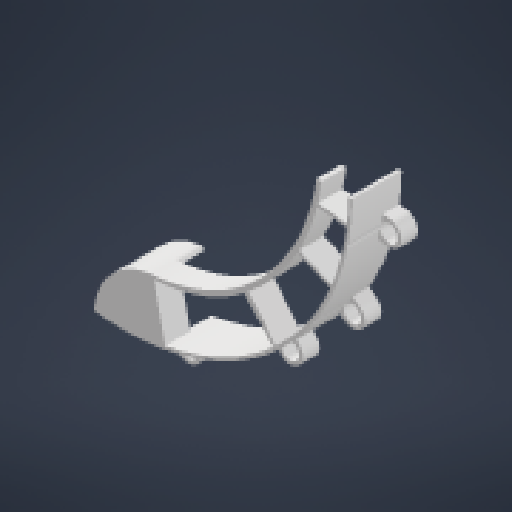
# Autodesk Inventor part: HalfFilterWall2
Saved by Autodesk Inventor 2026 (Build 300175050, 175E)
## iProperties
Created: 2026-05-05
Part Number: HalfFilterWall2
Material: Generic
Document SubType Name: Modeling
Designer: sniel
Density: 1 g/cm^3
Appearance: Default
Author: sniel
Autodesk Inventor part; units mm, degrees
ref_plane "YZ Plane" through (0, 0, 0) normal (1, 0, 0) x (0, 1, 0)
ref_plane "XZ Plane" through (0, 0, 0) normal (0, 1, 0) x (-1, 0, 0)
ref_plane "XY Plane" through (0, 0, 0) normal (0, 0, 1) x (1, 0, 0)
sketch "Sketch1" plane through (0, 0, 0) normal (0, 0, 1) x (1, 0, 0)
  arc A0 (23.689125, 20.041184) -> (18.254395, 20.887332) centre (0, -114.235526) ccw
  arc A1 (18.254395, 20.887332) -> (1.007395, 22.112112) centre (0, -114.119689) ccw
  arc A2 (1.007395, 22.112112) -> (0, 21.11214) centre (1, 21.11214) ccw
  line L0 (0, 21.11214) -> (0, 20.996303)
  arc A3 (0, 20.996303) -> (0.992605, 19.99633) centre (1, 20.996303) ccw
  arc A4 (16.894539, 18.932605) -> (0.992605, 19.99633) centre (0, -114.235526) ccw
  arc A5 (17.756944, 17.787789) -> (16.894539, 18.932605) centre (16.768682, 17.940556) ccw
  line L1 (17.756944, 17.787789) -> (16.790242, 11.534134)
  arc A6 (15.60857, 10.705783) -> (16.790242, 11.534134) centre (15.80198, 11.686902) ccw
  arc A7 (15.60857, 10.705783) -> (1.079217, 12.70838) centre (-9, -114.127341) ccw
  arc A8 (1.079217, 12.70838) -> (0, 11.711522) centre (1, 11.711522) ccw
  line L2 (0, 11.711522) -> (0, 11.060813)
  arc A9 (0, 11.060813) -> (0.916491, 10.064306) centre (1, 11.060813) ccw
  arc A10 (115.231581, -113.243479) -> (0.916491, 10.064306) centre (-9.5, -114.235526) ccw
  arc A11 (118.232397, -113.228461) -> (114.566766, -83.793446) centre (-9, -114.127341) ccw
  arc A12 (115.32455, -82.578069) -> (114.566766, -83.793446) centre (115.537931, -83.555038) ccw
  line L3 (115.32455, -82.578069) -> (128.714541, -79.65355)
  arc A13 (129.895591, -80.378296) -> (128.714541, -79.65355) centre (128.927921, -80.630519) ccw
  arc A14 (134.231856, -113.242921) -> (129.895591, -80.378296) centre (0, -114.235526) ccw
  arc A15 (134.231856, -113.242921) -> (135.231829, -114.235526) centre (135.231829, -113.235526) ccw
  line L4 (135.231829, -114.235526) -> (135.232636, -114.235526)
  arc A16 (135.232636, -114.235526) -> (136.232614, -113.228988) centre (135.232636, -113.235526) ccw
  arc A17 (136.232614, -113.228988) -> (135.007021, -95.865294) centre (0, -114.119689) ccw
  line L5 (135.007021, -95.865294) -> (135.104981, -95.849292)
  arc A18 (135.104981, -95.849292) -> (134.27671, -90.546401) centre (0, -114.235526) ccw
  arc A19 (133.568756, -86.834851) -> (134.27671, -90.546401) centre (138.734281, -87.772854) ccw
  arc A20 (133.568756, -86.834851) -> (132.332251, -81.378487) centre (0, -114.235526) ccw
  line L6 (132.332251, -81.378487) -> (132.247295, -81.397042)
  arc A21 (132.247295, -81.397042) -> (116.651364, -43.745136) centre (0, -114.119689) ccw
  line L7 (116.651364, -43.745136) -> (116.697607, -43.715472)
  arc A22 (116.697607, -43.715472) -> (113.822576, -39.163356) centre (0, -114.235526) ccw
  arc A23 (111.698714, -36.038295) -> (113.822576, -39.163356) centre (116.811886, -34.84751) ccw
  arc A24 (111.698714, -36.038295) -> (108.408382, -31.537085) centre (0, -114.235526) ccw
  line L8 (108.408382, -31.537085) -> (108.372186, -31.563116)
  arc A25 (108.372186, -31.563116) -> (82.556573, -5.747503) centre (0, -114.119689) ccw
  line L9 (82.556573, -5.747503) -> (82.569791, -5.729124)
  arc A26 (82.569791, -5.729124) -> (78.197231, -2.536812) centre (0, -114.235526) ccw
  arc A27 (75.07217, -0.41295) -> (78.197231, -2.536812) centre (79.388016, 2.57636) ccw
  arc A28 (75.07217, -0.41295) -> (70.382977, 2.544807) centre (0, -114.235526) ccw
  line L10 (70.382977, 2.544807) -> (70.374553, 2.531675)
  arc A29 (70.374553, 2.531675) -> (32.722647, 18.127606) centre (0, -114.119689) ccw
  line L11 (32.722647, 18.127606) -> (32.723148, 18.129897)
  arc A30 (32.723148, 18.129897) -> (27.400675, 19.33323) centre (0, -114.235526) ccw
  arc A31 (23.689125, 20.041184) -> (27.400675, 19.33323) centre (26.462672, 24.498755) ccw
  arc A32 (113.560126, -79.952698) -> (76.239267, -19.664872) centre (-9, -114.127341) ccw
  arc A33 (76.174631, -18.243916) -> (76.239267, -19.664872) centre (76.9092, -18.92245) ccw
  line L12 (76.174631, -18.243916) -> (83.492463, -10.321763)
  arc A34 (84.859198, -10.225464) -> (83.492463, -10.321763) centre (84.227031, -11.000297) ccw
  arc A35 (128.819481, -76.490091) -> (84.859198, -10.225464) centre (0, -114.235526) ccw
  arc A36 (128.073209, -77.748248) -> (128.819481, -76.490091) centre (127.859828, -76.771279) ccw
  line L13 (128.073209, -77.748248) -> (114.73676, -80.661074)
  arc A37 (113.560126, -79.952698) -> (114.73676, -80.661074) centre (114.52338, -79.684104) ccw
  line L14 (18.728755, 11.004204) -> (19.737656, 17.530849)
  arc A38 (20.881477, 18.365908) -> (19.737656, 17.530849) centre (20.725918, 17.378082) ccw
  arc A39 (81.689945, -7.718254) -> (20.881477, 18.365908) centre (0, -114.235526) ccw
  arc A40 (81.815957, -9.190298) -> (81.689945, -7.718254) centre (81.081388, -8.511764) ccw
  line L15 (81.815957, -9.190298) -> (74.632091, -16.967423)
  arc A41 (73.251075, -17.051848) -> (74.632091, -16.967423) centre (73.897522, -16.288889) ccw
  arc A42 (73.251075, -17.051848) -> (19.493078, 9.876833) centre (-9, -114.127341) ccw
  arc A43 (18.728755, 11.004204) -> (19.493078, 9.876833) centre (19.717017, 10.851436) ccw
  circle A44 centre (26.462672, -252.969807) radius 5.25
  circle A45 centre (79.388016, -231.047412) radius 5.25
  circle A46 centre (138.734281, -140.698198) radius 5.25
  circle A47 centre (116.811886, -193.623542) radius 5.25
  line L16 (70.374553, -230.886891) -> (73.075233, -235.096951)
  arc A48 (73.075233, -235.096951) -> (85.476933, -226.668474) centre (79.388016, -231.047412) ccw
  line L17 (85.476933, -226.668474) -> (82.556573, -222.607712)
  arc A49 (82.556573, -222.607712) -> (108.372186, -196.792099) centre (0, -114.235526) ccw
  line L18 (108.372186, -196.792099) -> (112.432948, -199.712459)
  arc A50 (112.432948, -199.712459) -> (120.861425, -187.310759) centre (116.811886, -193.623542) ccw
  line L19 (120.861425, -187.310759) -> (116.651364, -184.610079)
  arc A51 (116.651364, -184.610079) -> (132.247295, -146.958173) centre (0, -114.235526) ccw
  line L20 (132.247295, -146.958173) -> (137.133926, -148.025467)
  arc A52 (137.133926, -148.025467) -> (139.943419, -133.296307) centre (138.734281, -140.698198) ccw
  line L21 (139.943419, -133.296307) -> (135.007021, -132.489921)
  arc A53 (135.007021, -132.489921) -> (136.235526, -114.235526) centre (0, -114.235526) ccw
  line L22 (136.235526, -114.235526) -> (134.235526, -114.235526)
  line L23 (0, -248.471052) -> (0, -250.471052)
  arc A54 (19.060781, -254.178945) -> (33.789941, -251.369452) centre (26.462672, -252.969807) ccw
  line L24 (33.789941, -251.369452) -> (32.722647, -246.482821)
  arc A55 (32.722647, -246.482821) -> (70.374553, -230.886891) centre (0, -114.235526) ccw
  arc A56 (69.722359, -193.081889) -> (115.100471, -114.235526) centre (-4.40842, -97.9364) ccw
  line L25 (118.110658, -114.235526) -> (115.100471, -114.235526)
  line L26 (133.484281, -128.417314) -> (112.842728, -126.224291)
  line L27 (133.484281, -128.417314) -> (133.258174, -130.404492)
  line L28 (115.9197, -126.551198) -> (115.452307, -128.495817)
  line L29 (115.452307, -128.495817) -> (133.258174, -130.404492)
  line L30 (124.355241, -164.782045) -> (123.588357, -166.629175)
  line L31 (123.588357, -166.629175) -> (103.639403, -158.346853)
  line L32 (124.355241, -164.782045) -> (104.606006, -156.582642)
  line L33 (89.213784, -214.535462) -> (90.698228, -213.195154)
  line L34 (90.698228, -213.195154) -> (72.751914, -190.641952)
  line L35 (89.213784, -214.535462) -> (69.722359, -193.081889)
  circle A57 centre (-138.734281, -140.698198) radius 5.25
  circle A58 centre (-116.811886, -193.623542) radius 5.25
  circle A59 centre (-26.462672, -252.969807) radius 5.25
  circle A60 centre (-79.388016, -231.047412) radius 5.25
  line L36 (-116.651364, -184.610079) -> (-120.861425, -187.310759)
  arc A61 (-120.861425, -187.310759) -> (-112.432948, -199.712459) centre (-116.811886, -193.623542) ccw
  line L37 (-112.432948, -199.712459) -> (-108.372186, -196.792099)
  arc A62 (-108.372186, -196.792099) -> (-82.556573, -222.607712) centre (0, -114.235526) ccw
  line L38 (-82.556573, -222.607712) -> (-85.476933, -226.668474)
  arc A63 (-85.476933, -226.668474) -> (-73.075233, -235.096951) centre (-79.388016, -231.047412) ccw
  line L39 (-73.075233, -235.096951) -> (-70.374553, -230.886891)
  arc A64 (-70.374553, -230.886891) -> (-32.722647, -246.482821) centre (0, -114.235526) ccw
  line L40 (-32.722647, -246.482821) -> (-33.789941, -251.369452)
  arc A65 (-33.789941, -251.369452) -> (-19.060781, -254.178945) centre (-26.462672, -252.969807) ccw
  line L41 (-19.060781, -254.178945) -> (-18.254395, -249.242547)
  arc A66 (-18.254395, -249.242547) -> (0, -250.471052) centre (0, -114.235526) ccw
  line L42 (0, -250.471052) -> (0, -248.471052)
  arc A67 (-134.235526, -114.235526) -> (0, -248.471052) centre (0, -114.235526) ccw
  line L43 (-134.235526, -114.235526) -> (-136.235526, -114.235526)
  arc A68 (-136.235526, -114.235526) -> (-135.007021, -132.489921) centre (0, -114.235526) ccw
  line L44 (-135.007021, -132.489921) -> (-139.943419, -133.296307)
  arc A69 (-139.943419, -133.296307) -> (-137.133926, -148.025467) centre (-138.734281, -140.698198) ccw
  line L45 (-137.133926, -148.025467) -> (-132.247295, -146.958173)
  arc A70 (-132.247295, -146.958173) -> (-116.651364, -184.610079) centre (0, -114.235526) ccw
  arc A71 (22.567907, -246.560376) -> (27.724702, -245.576751) centre (26.462672, -252.969807) ccw
  arc A72 (22.567907, -246.560376) -> (134.235526, -114.235526) centre (0, -114.235526) ccw
  line L46 (0, -248.471052) -> (0, -216.471052)
  line L47 (0, -216.471052) -> (0, -214.471052)
  circle A73 centre (0, -250.471052) radius 16
  line L48 (26.462672, -252.969807) -> (22.567907, -246.560376)
  circle A74 centre (22.567907, -246.560376) radius 32
  arc A75 (16.034625, -215.234409) -> (-15.97239, -249.531503) centre (24.34296, -255.071453) ccw
  line L49 (22.567907, -246.560376) -> (16.034625, -215.234409)
  line L50 (16.034625, -215.234409) -> (15.626295, -213.276536)
  arc A76 (15.626295, -213.276536) -> (-18.254395, -249.242547) centre (20.539292, -251.84582) ccw
  arc A77 (71.73985, -195.302476) -> (118.110658, -114.235526) centre (-2.270449, -99.172443) ccw
  arc A78 (15.626295, -213.276536) -> (69.722359, -193.081889) centre (7.954113, -110.173035) ccw
  arc A79 (16.034625, -215.234409) -> (71.73985, -195.302476) centre (13.040909, -119.059964) ccw
  line L51 (15.626295, -213.276536) -> (17.619252, -213.108837)
  line L52 (22.567907, -246.560376) -> (24.53688, -246.209455)
  line L53 (24.53688, -246.209455) -> (17.619252, -213.108837)
  point P0 (74.632091, -193.004777)
  point P1 (33.789941, -244.148637)
  point P2 (36.843345, -243.315905)
  point P3 (33.789941, -251.369452)
  point P4 (-15.213711, -245.516964)
  point P5 (24.373197, -214.61134)
  point P6 (19.060781, -254.178945)
  point P7 (33.789941, -251.369452)
  point P8 (18.045983, -215.150731)
  point P9 (17.991354, -214.88933)
  point P10 (22.567907, -246.560376)
  dimension "d68" = 32
  dimension "d69" = 64
  dimension "d54" = 2
  dimension "d55" = 2
  dimension "d56" = 2
  dimension "d57" = 2
  dimension "d66" = 32
  dimension "d67" = 2
  dimension "d70" = 2
  dimension "d71" = 2
  dimension "d72" = 2
  constraints: 148 point on circle, 108 end point, 77 centre point, 4 point on line, 3 coincident, 1 concentric, 1 horizontal, 1 perpendicular, 1 tangent, 21 other
  measures "d54" distance of L26.start L27.end
  measures "d55" distance of L28.start L28.end
  measures "d56" distance of L30.start L30.end
  measures "d57" distance of L33.start L33.end
  measures "d66" distance of L23.start L46.end
  measures "d67" distance of L46.end L47.end
  measures "d70" distance of L49.end L50.end
  measures "d71" distance of L50.end L51.end
  measures "d72" distance of L49.start L52.end
extrude "Extrusion1" add sketch "Sketch1" along normal blind 30 contours A55 A74 A72 L22 A53 L21 A52 L20 A51 L19 A50 L18 A49 L17 A48 L16 | A55 L24 A71 A72 A74 | A54 A71 A72 | L35 A77 L34 L33 | A74 L53 A78 L35 A79 | A66 A76 A67 A73 | A72 L52 | L52 L49 A79 L53 | L35 A56 L34 A77 | L53 A79 A74 | A74 L50 A78 L53 | A67 A76 L46 A75 A73 | L34 A56 L26 L28 A77 | L31 A77 L32 L30 | A75 L46 A76 L50 | A56 L25 A77 L26 | L29 A77 L26 L27 | A77 L28 picked at (17.804356, -215.074453)
sketch "Sketch9" plane through (0, 0, 0) normal (0, 0, -1) x (-1, 0, 0)
  line L0 (-136.235526, -114.235526) -> (-134.235526, -114.235526)
  arc A0 (-134.235526, -114.235526) -> (-133.484281, -128.417314) centre (0, -114.235526) ccw
  arc A1 (-90.698228, -213.195154) -> (-89.213784, -214.535462) centre (0, -114.235526) ccw
  line L1 (-71.73985, -195.302476) -> (-89.213784, -214.535462)
  line L2 (-89.213784, -214.535462) -> (-90.698228, -213.195154)
  line L3 (-90.698228, -213.195154) -> (-74.632091, -193.004777)
  line L4 (-115.452307, -128.495817) -> (-133.258174, -130.404492)
  line L5 (-133.258174, -130.404492) -> (-133.484281, -128.417314)
  line L6 (-133.484281, -128.417314) -> (-115.9197, -126.551198)
  line L7 (-118.110658, -114.235526) -> (-115.100471, -114.235526)
  arc A2 (-115.100471, -114.235526) -> (-69.722359, -193.081889) centre (4.40842, -97.9364) ccw
  line L8 (-33.789941, -251.369452) -> (-32.722647, -246.482821)
  arc A3 (-70.374553, -230.886891) -> (-32.722647, -246.482821) centre (0, -114.235526) ccw
  line L9 (-70.374553, -230.886891) -> (-73.075233, -235.096951)
  arc A4 (-85.476933, -226.668474) -> (-73.075233, -235.096951) centre (-79.388016, -231.047412) ccw
  line L10 (-85.476933, -226.668474) -> (-82.556573, -222.607712)
  arc A5 (-108.372186, -196.792099) -> (-82.556573, -222.607712) centre (0, -114.235526) ccw
  line L11 (-108.372186, -196.792099) -> (-112.432948, -199.712459)
  arc A6 (-120.861425, -187.310759) -> (-112.432948, -199.712459) centre (-116.811886, -193.623542) ccw
  line L12 (-120.861425, -187.310759) -> (-116.651364, -184.610079)
  arc A7 (-132.247295, -146.958173) -> (-116.651364, -184.610079) centre (0, -114.235526) ccw
  line L13 (-132.247295, -146.958173) -> (-137.133926, -148.025467)
  arc A8 (-139.943419, -133.296307) -> (-137.133926, -148.025467) centre (-138.734281, -140.698198) ccw
  line L14 (-139.943419, -133.296307) -> (-135.007021, -132.489921)
  arc A9 (-136.235526, -114.235526) -> (-135.007021, -132.489921) centre (0, -114.235526) ccw
  circle A10 centre (-116.811886, -193.623542) radius 5.25
  circle A11 centre (-138.734281, -140.698198) radius 5.25
  circle A12 centre (-79.388016, -231.047412) radius 5.25
  circle A13 centre (0, -114.235526) radius 134.235526
  arc A14 (-118.110658, -114.235526) -> (-115.9197, -126.551198) centre (2.270449, -99.172443) ccw
  arc A15 (-103.639403, -158.346853) -> (-74.632091, -193.004777) centre (2.270449, -99.172443) ccw
  arc A16 (-133.258174, -130.404492) -> (-124.355241, -164.782045) centre (0, -114.235526) ccw
  arc A17 (-89.213784, -214.535462) -> (-24.53688, -246.209455) centre (0, -114.235526) ccw
  arc A18 (-133.484281, -128.417314) -> (-133.258174, -130.404492) centre (0, -114.235526) ccw
  arc A19 (-124.355241, -164.782045) -> (-123.588357, -166.629175) centre (0, -114.235526) ccw
  arc A20 (-33.789941, -251.369452) -> (-22.567907, -246.560376) centre (-26.462672, -252.969807) ccw
  arc A21 (-69.722359, -193.081889) -> (-15.626295, -213.276536) centre (-7.954113, -110.173035) ccw
  arc A22 (18.254395, -249.242547) -> (-15.626295, -213.276536) centre (-20.539292, -251.84582) ccw
  arc A23 (15.97239, -249.531503) -> (18.254395, -249.242547) centre (0, -114.235526) ccw
  arc A24 (15.97239, -249.531503) -> (15.213711, -245.516964) centre (0, -250.471052) ccw
  arc A25 (15.213711, -245.516964) -> (-16.034625, -215.234409) centre (-24.34296, -255.071453) ccw
  arc A26 (-17.991354, -214.88933) -> (-24.373197, -214.61134) centre (-22.567907, -246.560376) ccw
  arc A27 (-71.73985, -195.302476) -> (-24.373197, -214.61134) centre (-13.040909, -119.059964) ccw
  line L15 (-103.639403, -158.346853) -> (-123.588357, -166.629175)
  line L16 (-123.588357, -166.629175) -> (-124.355241, -164.782045)
  line L17 (-124.355241, -164.782045) -> (-104.606006, -156.582642)
  arc A28 (-115.452307, -128.495817) -> (-104.606006, -156.582642) centre (2.270449, -99.172443) ccw
  circle A29 centre (-24.34296, -255.071453) radius 40.460125
  arc A30 (-71.73985, -195.302476) -> (-24.373197, -214.61134) centre (-13.040909, -119.059964) ccw
  arc A31 (-69.722359, -193.081889) -> (-15.626295, -213.276536) centre (-7.954113, -110.173035) ccw
  line L18 (-24.373197, -214.61134) -> (-15.626295, -213.276536)
  line L19 (-16.034625, -215.234409) -> (-22.567907, -246.560376)
  arc A32 (-123.588357, -166.629175) -> (-90.698228, -213.195154) centre (0, -114.235526) ccw
  line L20 (-24.53688, -246.209455) -> (-17.991354, -214.88933)
  point P0 (0, 0)
  point P1 (-24.53688, -246.209455)
  point P2 (-133.484281, -128.417314)
  point P3 (-133.258174, -130.404492)
  point P4 (-124.355241, -164.782045)
  point P5 (-22.567907, -246.560376)
  point P6 (-89.213784, -214.535462)
  point P7 (-90.698228, -213.195154)
  point P8 (-133.484281, -128.417314)
  point P9 (-124.355241, -164.782045)
  point P10 (15.730389, -247.546183)
  point P11 (18.068997, -247.249389)
  point P12 (-22.567907, -246.560376)
  point P13 (-24.53688, -246.209455)
  point P14 (15.418073, -247.582665)
  point P15 (-18.036598, -215.105825)
  constraints: 2 coincident, 2 end point, 1 centre point, 3 other
extrude "Extrusion8" cut sketch "Sketch9" against normal blind 15 contours A13 A22 A21 A2 L7 A14 L6 A0 | L6 A14 L7 A2 A21 L18 A27 L1 L2 L3 A15 L15 L16 L17 A28 L4 L5 | L4 A28 L17 A13 | L16 A13 | A13 A29 L19 A25 A24 | L15 A15 L3 A13 | A13 L19 A29 | A29 A13 L1 A27 | A26 L20 A29 | A29 L20 A13 | A13 L20 A29 L19
sketch "Sketch10" plane through (0, 0, 30) normal (0, 0, 1) x (1, 0, 0)
  line L0 (136.235526, -114.235526) -> (134.235526, -114.235526)
  line L1 (71.73985, -195.302476) -> (89.213784, -214.535462)
  line L2 (89.213784, -214.535462) -> (90.698228, -213.195154)
  line L3 (90.698228, -213.195154) -> (74.632091, -193.004777)
  line L4 (115.452307, -128.495817) -> (133.258174, -130.404492)
  line L5 (133.258174, -130.404492) -> (133.484281, -128.417314)
  line L6 (133.484281, -128.417314) -> (115.9197, -126.551198)
  arc A0 (115.9197, -126.551198) -> (118.110658, -114.235526) centre (-2.270449, -99.172443) ccw
  line L7 (118.110658, -114.235526) -> (115.100471, -114.235526)
  arc A1 (69.722359, -193.081889) -> (115.100471, -114.235526) centre (-4.40842, -97.9364) ccw
  line L8 (33.789941, -251.369452) -> (32.722647, -246.482821)
  arc A2 (32.722647, -246.482821) -> (70.374553, -230.886891) centre (0, -114.235526) ccw
  line L9 (70.374553, -230.886891) -> (73.075233, -235.096951)
  arc A3 (73.075233, -235.096951) -> (85.476933, -226.668474) centre (79.388016, -231.047412) ccw
  line L10 (85.476933, -226.668474) -> (82.556573, -222.607712)
  arc A4 (82.556573, -222.607712) -> (108.372186, -196.792099) centre (0, -114.235526) ccw
  line L11 (108.372186, -196.792099) -> (112.432948, -199.712459)
  arc A5 (112.432948, -199.712459) -> (120.861425, -187.310759) centre (116.811886, -193.623542) ccw
  line L12 (120.861425, -187.310759) -> (116.651364, -184.610079)
  arc A6 (116.651364, -184.610079) -> (132.247295, -146.958173) centre (0, -114.235526) ccw
  line L13 (132.247295, -146.958173) -> (137.133926, -148.025467)
  arc A7 (137.133926, -148.025467) -> (139.943419, -133.296307) centre (138.734281, -140.698198) ccw
  line L14 (139.943419, -133.296307) -> (135.007021, -132.489921)
  arc A8 (135.007021, -132.489921) -> (136.235526, -114.235526) centre (0, -114.235526) ccw
  circle A9 centre (116.811886, -193.623542) radius 5.25
  circle A10 centre (138.734281, -140.698198) radius 5.25
  circle A11 centre (79.388016, -231.047412) radius 5.25
  circle A12 centre (0, -114.235526) radius 136.235526
  arc A13 (74.632091, -193.004777) -> (103.639403, -158.346853) centre (-2.270449, -99.172443) ccw
  arc A14 (133.484281, -128.417314) -> (134.235526, -114.235526) centre (0, -114.235526) ccw
  arc A15 (124.355241, -164.782045) -> (133.258174, -130.404492) centre (0, -114.235526) ccw
  arc A16 (89.213784, -214.535462) -> (90.698228, -213.195154) centre (0, -114.235526) ccw
  arc A17 (24.53688, -246.209455) -> (89.213784, -214.535462) centre (0, -114.235526) ccw
  arc A18 (133.258174, -130.404492) -> (133.484281, -128.417314) centre (0, -114.235526) ccw
  arc A19 (123.588357, -166.629175) -> (124.355241, -164.782045) centre (0, -114.235526) ccw
  arc A20 (22.567907, -246.560376) -> (33.789941, -251.369452) centre (26.462672, -252.969807) ccw
  arc A21 (15.626295, -213.276536) -> (69.722359, -193.081889) centre (7.954113, -110.173035) ccw
  arc A22 (15.626295, -213.276536) -> (-18.254395, -249.242547) centre (20.539292, -251.84582) ccw
  arc A23 (-18.254395, -249.242547) -> (-15.97239, -249.531503) centre (0, -114.235526) ccw
  arc A24 (-15.213711, -245.516964) -> (-15.97239, -249.531503) centre (0, -250.471052) ccw
  arc A25 (16.034625, -215.234409) -> (-15.213711, -245.516964) centre (24.34296, -255.071453) ccw
  arc A26 (24.373197, -214.61134) -> (17.991354, -214.88933) centre (22.567907, -246.560376) ccw
  arc A27 (24.373197, -214.61134) -> (71.73985, -195.302476) centre (13.040909, -119.059964) ccw
  line L15 (103.639403, -158.346853) -> (123.588357, -166.629175)
  line L16 (123.588357, -166.629175) -> (124.355241, -164.782045)
  line L17 (124.355241, -164.782045) -> (104.606006, -156.582642)
  arc A28 (104.606006, -156.582642) -> (115.452307, -128.495817) centre (-2.270449, -99.172443) ccw
  line L18 (16.034625, -215.234409) -> (22.567907, -246.560376)
  arc A29 (90.698228, -213.195154) -> (123.588357, -166.629175) centre (0, -114.235526) ccw
  line L19 (24.53688, -246.209455) -> (17.991354, -214.88933)
  point P0 (0, 0)
  point P1 (134.108488, -138.215349)
  point P2 (133.519349, -141.303992)
  point P3 (132.247295, -146.958173)
  point P4 (113.552733, -189.507667)
  point P5 (111.785317, -192.108252)
  point P6 (108.372186, -196.792099)
  point P7 (77.872726, -226.020843)
  point P8 (75.272141, -227.78826)
  point P9 (70.374553, -230.886891)
  point P10 (20.113116, -248.978174)
  constraints: 1 coincident, 3 other
extrude "Extrusion9" cut sketch "Sketch10" against normal blind 20 contours A19 L16 | A18 L5 | L14 A7 L13 A12 A10 | A12 A10 | A12 L8 A20 | L12 A5 L11 A12 A9 | A12 A11 L10 A3 L9 | A12 A9 | A11 A12 picked at (133.709166, -139.561852) picked at (112.651459, -190.584808) picked at (76.638241, -226.690601)
sketch "Sketch12" plane through (0, 0, 30) normal (0, 0, 1) x (1, 0, 0)
  arc A0 (20.113116, -248.978174) -> (23.979823, -248.344014) centre (0, -114.235526) ccw
  arc A1 (27.068466, -247.754876) -> (23.979823, -248.344014) centre (26.462672, -252.969807) ccw
  arc A2 (27.068466, -247.754876) -> (75.272141, -227.78826) centre (0, -114.235526) ccw
  arc A3 (77.872726, -226.020843) -> (75.272141, -227.78826) centre (79.388016, -231.047412) ccw
  arc A4 (77.872726, -226.020843) -> (111.785317, -192.108252) centre (0, -114.235526) ccw
  arc A5 (113.552733, -189.507667) -> (111.785317, -192.108252) centre (116.811886, -193.623542) ccw
  arc A6 (113.552733, -189.507667) -> (133.519349, -141.303992) centre (0, -114.235526) ccw
  arc A7 (134.108488, -138.215349) -> (133.519349, -141.303992) centre (138.734281, -140.698198) ccw
  arc A8 (134.108488, -138.215349) -> (136.235526, -114.235526) centre (0, -114.235526) ccw
  line L0 (136.235526, -114.235526) -> (134.235526, -114.235526)
  arc A9 (133.484281, -128.417314) -> (134.235526, -114.235526) centre (0, -114.235526) ccw
  arc A10 (133.258174, -130.404492) -> (133.484281, -128.417314) centre (0, -114.235526) ccw
  arc A11 (124.355241, -164.782045) -> (133.258174, -130.404492) centre (0, -114.235526) ccw
  arc A12 (123.588357, -166.629175) -> (124.355241, -164.782045) centre (0, -114.235526) ccw
  arc A13 (90.698228, -213.195154) -> (123.588357, -166.629175) centre (0, -114.235526) ccw
  arc A14 (89.213784, -214.535462) -> (90.698228, -213.195154) centre (0, -114.235526) ccw
  arc A15 (24.53688, -246.209455) -> (89.213784, -214.535462) centre (0, -114.235526) ccw
  line L1 (24.53688, -246.209455) -> (17.991354, -214.88933)
  arc A16 (24.373197, -214.61134) -> (17.991354, -214.88933) centre (22.567907, -246.560376) ccw
  arc A17 (24.373197, -214.61134) -> (71.73985, -195.302476) centre (13.040909, -119.059964) ccw
  line L2 (71.73985, -195.302476) -> (89.213784, -214.535462)
  line L3 (89.213784, -214.535462) -> (90.698228, -213.195154)
  line L4 (90.698228, -213.195154) -> (74.632091, -193.004777)
  arc A18 (74.632091, -193.004777) -> (103.639403, -158.346853) centre (-2.270449, -99.172443) ccw
  line L5 (103.639403, -158.346853) -> (123.588357, -166.629175)
  line L6 (123.588357, -166.629175) -> (124.355241, -164.782045)
  line L7 (124.355241, -164.782045) -> (104.606006, -156.582642)
  arc A19 (104.606006, -156.582642) -> (115.452307, -128.495817) centre (-2.270449, -99.172443) ccw
  line L8 (115.452307, -128.495817) -> (133.258174, -130.404492)
  line L9 (133.258174, -130.404492) -> (133.484281, -128.417314)
  line L10 (133.484281, -128.417314) -> (115.9197, -126.551198)
  arc A20 (115.9197, -126.551198) -> (118.110658, -114.235526) centre (-2.270449, -99.172443) ccw
  line L11 (118.110658, -114.235526) -> (115.100471, -114.235526)
  arc A21 (69.722359, -193.081889) -> (115.100471, -114.235526) centre (-4.40842, -97.9364) ccw
  arc A22 (15.626295, -213.276536) -> (69.722359, -193.081889) centre (7.954113, -110.173035) ccw
  arc A23 (15.626295, -213.276536) -> (-18.254395, -249.242547) centre (20.539292, -251.84582) ccw
  arc A24 (-18.254395, -249.242547) -> (-15.97239, -249.531503) centre (0, -114.235526) ccw
  arc A25 (-15.213711, -245.516964) -> (-15.97239, -249.531503) centre (0, -250.471052) ccw
  arc A26 (16.034625, -215.234409) -> (-15.213711, -245.516964) centre (24.34296, -255.071453) ccw
  line L12 (16.034625, -215.234409) -> (22.567907, -246.560376)
  arc A27 (22.567907, -246.560376) -> (20.113116, -248.978174) centre (26.462672, -252.969807) ccw
  circle A28 centre (0, -114.235526) radius 136.235526
  point P0 (0, 0)
  point P1 (20.113116, -248.978174)
  constraints: 1 coincident, 3 other
extrude "Extrusion11" add sketch "Sketch12" against normal blind 2 contours A28 A25 A26 L12 A27
sketch "Sketch13" plane through (0, 0, 10) normal (0, 0, 1) x (1, 0, 0)
  arc A0 (23.979823, -248.344014) -> (27.068466, -247.754876) centre (26.462672, -252.969807) ccw
  arc A1 (20.113116, -248.978174) -> (23.979823, -248.344014) centre (0, -114.235526) ccw
  arc A2 (20.113116, -248.978174) -> (33.789941, -251.369452) centre (26.462672, -252.969807) ccw
  line L0 (32.722647, -246.482821) -> (33.789941, -251.369452)
  arc A3 (27.068466, -247.754876) -> (32.722647, -246.482821) centre (0, -114.235526) ccw
  point P0 (0, 0)
extrude "Extrusion12" add sketch "Sketch13" along normal blind 8
fillet "Fillet3" radius 2 1 edges at (24.3732, -214.6113, 7.5)
body "Solid1"
